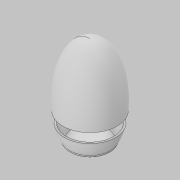
# Autodesk Inventor part: 메인 형상
Saved by Autodesk Inventor 2021 (Build 250183000, 183)
## iProperties
Created: 2022-06-02
Part Number: 메인 형상
Material: 일반
Document SubType Name: Modeling
Designer: fly01
Density: 1 g/cm^3
Appearance: 기본값
Author: fly01
Autodesk Inventor part; units mm, degrees
ref_plane "YZ Plane" through (0, 0, 0) normal (1, 0, 0) x (0, 1, 0)
ref_plane "XZ Plane" through (0, 0, 0) normal (0, 1, 0) x (-1, 0, 0)
ref_plane "XY Plane" through (0, 0, 0) normal (0, 0, 1) x (1, 0, 0)
sketch "스케치1" plane through (0, 0, 0) normal (0, 0, 1) x (1, 0, 0)
  line L0 (-24.5, -42.5) -> (24.5, -42.5)
  line L1 (28, -39) -> (28, 39)
  line L2 (24.5, 42.5) -> (-24.5, 42.5)
  line L3 (-28, 39) -> (-28, -39)
  line L4 (-28, -42.5) -> (28, 42.5) construction
  line L5 (28, -42.5) -> (-28, 42.5) construction
  arc A0 (-24.5, 42.5) -> (-28, 39) centre (-24.5, 39) ccw
  arc A1 (28, 39) -> (24.5, 42.5) centre (24.5, 39) ccw
  arc A2 (24.5, -42.5) -> (28, -39) centre (24.5, -39) ccw
  arc A3 (-28, -39) -> (-24.5, -42.5) centre (-24.5, -39) ccw
  circle A4 centre (-24.5, 39) radius 1.35
  circle A5 centre (24.5, 39) radius 1.35
  circle A6 centre (-24.5, -39) radius 1.35
  circle A7 centre (24.5, -39) radius 1.35
  point P0 (0, 0)
  dimension "d1" = 56
  dimension "d2" = 85
  dimension "d3" = 3.5
  dimension "d4" = 2.7
  dimension "d5" = 2.7
  dimension "d6" = 2.7
  dimension "d7" = 2.7
  constraints: 12 end point, 8 centre point, 8 point on circle, 8 point on line, 8 tangent, 4 coincident, 3 equal radius, 2 parallel, 1 horizontal, 1 perpendicular
  measures "d1" distance of L5.end L4.end
  measures "d2" distance of L4.end L5.start
  measures "d3" radius of A0
  measures "d4" diameter of A4
  measures "d5" diameter of A5
  measures "d6" diameter of A6
  measures "d7" diameter of A7
sketch "스케치2" plane through (0, 0, 0) normal (0, 0, 1) x (1, 0, 0)
  circle A0 centre (0, 0) radius 50
  circle A1 centre (0, 0) radius 55
  dimension "d8" = 100
  dimension "d9" = 110
  constraints: 2 centre point, 2 coincident
  measures "d8" diameter of A0
  measures "d9" diameter of A1
sketch "스케치3" plane through (0, 0, 0) normal (1, 0, 0) x (0, 1, 0)
  line L0 (0, 0) -> (0, 40)
  line L1 (0, 40) -> (75, 40) construction
  line L2 (75, 40) -> (70, 40) construction
  line L3 (50, 0) -> (-50, 0) projected
  line L4 (55, 0) -> (-55, 0) projected
  line L5 (55, 0) -> (75, 40) construction
  line L6 (50, 0) -> (70, 40) construction
  line L7 (0, 40) -> (0, 70)
  line L8 (0, 240) -> (54.7563, 240) construction
  line L9 (54.7563, 240) -> (84.2775, 163.091) construction
  line L10 (84.2775, 163.091) -> (81.4992, 39.6647) construction
  line L11 (81.4992, 39.6647) -> (50, 0) construction
  spline S0 degree 4 poles (0, 240) (54.7563, 240) (84.2775, 163.091) (81.4992, 39.6647) (50, 0) knots 1 1 1 1 1 2 2 2 2 2
  line L12 (0, 245) -> (0, 0) construction
  line L13 (71.2551, 70) -> (76.2766, 70)
  line L14 (66.6024, 40) -> (71.7254, 40)
  line L15 (56.2073, 0) -> (50, 0)
  line L16 (50, 0) -> (56.2073, 0)
  line L17 (0, 245) -> (0, 240)
  spline S1 degree 5 poles (0, 245) (5.1528, 244.9992) (10.3055, 244.4204) (15.3717, 243.1831) (25.1769, 239.3964) (33.8134, 233.3951) (37.8173, 229.8886) (45.5689, 221.7276) (51.8605, 212.3819) (54.8235, 207.2226) (60.4769, 195.8827) (64.8789, 183.9976) (66.9186, 177.5881) (70.6356, 164.0308) (73.3192, 150.2301) (74.4707, 142.9862) (76.3457, 128.1838) (77.3134, 113.2942) (77.5823, 105.7109) (77.678, 90.7476) (76.8875, 75.8052) (76.2754, 68.4532) (74.657, 54.5053) (72.0429, 40.7106) (70.548, 34.215) (67.267, 22.422) (62.6613, 11.084) (60.2333, 6.0681) (57.374, 1.2456) (53.9155, -3.1095) knots 0 0 0 0 0 0 0.08946 0.08946 0.08946 0.181234 0.181234 0.181234 0.284285 0.284285 0.284285 0.400927 0.400927 0.400927 0.528185 0.528185 0.528185 0.659854 0.659854 0.659854 0.78786 0.78786 0.78786 0.903467 0.903467 0.903467 1 1 1 1 1 1
  dimension "d16" = 5
  dimension "d11" = 40
  dimension "d12" = 75
  dimension "d13" = 5
  dimension "d14" = 30
  dimension "d15" = 170
  dimension "d17" = 30
  constraints: 24 end point, 3 point on line, 2 perpendicular, 2 vertical, 1 collinear, 1 horizontal, 11 other
  measures "d11" distance of L0.start L0.end
  measures "d12" distance of L0.end L1.end
  measures "d13" distance of L1.end L2.end
  measures "d14" distance of L0.end L7.end
  measures "d15" distance of L7.end L8.start
  measures "d17" distance between parallel lines of L14 L13
revolve "회전1" add sketch "스케치3" angle 360 about axis through (0, 0, 245) along (0, 0, -1) contours L4 S0 L14 S1 L15 | S0 L17 S1 L13
sketch "스케치4" plane through (0, 0, 0) normal (0, 0, -1) x (-1, 0, 0)
  circle A0 centre (0, 0) radius 56.2073 projected
  point P0 (0, 0)
  point P1 (0, 56.2073)
  constraints: 1 vertical alignment
extrude "돌출1" add sketch "스케치4" along normal blind 5
fillet "모깎기1" radius 2 1 edges at (56.2073, 0, -5)
